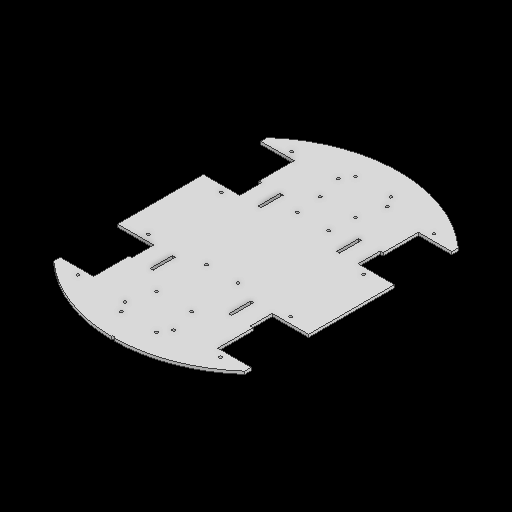
# Autodesk Inventor part: ChasisInferior
Saved by Autodesk Inventor 2025.2 (Build 292293000, 293)
## iProperties
Created: 2024-12-02
Part Number: ChasisInferior
Material: Generic
Document SubType Name: Modeling
Designer: braughton
Density: 1 g/cm^3
Appearance: Default
Author: braughton
Autodesk Inventor part; units mm, degrees
ref_plane "YZ Plane" through (0, 0, 0) normal (1, 0, 0) x (0, 1, 0)
ref_plane "XZ Plane" through (0, 0, 0) normal (0, 1, 0) x (-1, 0, 0)
ref_plane "XY Plane" through (0, 0, 0) normal (0, 0, 1) x (1, 0, 0)
sketch "Sketch1" plane through (0, 0, 0) normal (0, 1, 0) x (-1, 0, 0)
  circle A0 centre (-19.704, -123.7953) radius 1.5
  circle A1 centre (-26.6684, -112.9171) radius 1.5
  circle A2 centre (-75.7396, -112.9171) radius 1.5
  line L0 (-101.204, -106.1137) -> (-89.704, -106.1137)
  line L1 (-101.204, -106.1137) -> (-66.204, -106.1137)
  arc A3 (-101.204, -112.9171) -> (-1.204, -151.1137) centre (-1.204, -1.1137) ccw
  line L2 (-101.204, -106.1137) -> (-101.204, -112.9171)
  line L3 (-89.704, -106.1137) -> (-78.204, -106.1137)
  circle A4 centre (17.296, 121.5679) radius 1.5
  circle A5 centre (17.296, 84.5679) radius 1.5
  line L4 (63.796, 103.8863) -> (63.796, 66.8863)
  circle A6 centre (24.2604, 110.6897) radius 1.5
  circle A7 centre (73.3316, 110.6897) radius 1.5
  line L5 (98.796, 103.8863) -> (63.796, 103.8863)
  arc A8 (98.796, 110.6897) -> (-1.204, 148.8863) centre (-1.204, -1.1137) ccw
  line L6 (75.796, 43.8863) -> (87.296, 43.8863)
  circle A9 centre (73.3316, 37.0829) radius 1.5
  line L7 (87.296, 43.8863) -> (98.796, 43.8863)
  circle A10 centre (-19.704, 121.5679) radius 1.5
  circle A11 centre (-1.204, 148.8863) radius 1.5
  circle A12 centre (-26.6684, 110.6897) radius 1.5
  circle A13 centre (-75.7396, 110.6897) radius 1.5
  line L8 (-101.204, 103.8863) -> (-66.204, 103.8863)
  line L9 (-101.204, 103.8863) -> (-101.204, 110.6897)
  arc A14 (-1.204, 148.8863) -> (-101.204, 110.6897) centre (-1.204, -1.1137) ccw
  line L10 (-2.704, 148.8863) -> (-1.204, 148.8863)
  line L11 (0.296, 148.8863) -> (-1.204, 148.8863)
  line L12 (63.796, -69.1137) -> (60.796, -69.1137)
  line L13 (38.396, -69.1137) -> (41.396, -69.1137)
  line L14 (63.796, -46.1137) -> (98.796, -46.1137)
  line L15 (60.796, -69.1137) -> (60.796, -57.6137)
  line L16 (41.396, -69.1137) -> (41.396, -57.6137)
  line L17 (63.796, -46.1137) -> (60.796, -46.1137)
  line L18 (60.796, -46.1137) -> (60.796, -57.6137)
  line L19 (41.396, -46.1137) -> (41.396, -57.6137)
  line L20 (38.396, -46.1137) -> (41.396, -46.1137)
  line L21 (38.396, -57.6137) -> (38.396, -46.1137)
  circle A15 centre (73.3316, -39.3103) radius 1.5
  line L22 (38.396, -57.6137) -> (38.396, -69.1137)
  circle A16 centre (17.296, -123.7953) radius 1.5
  circle A17 centre (17.296, -86.7953) radius 1.5
  circle A18 centre (15.296, -60.7953) radius 1.5
  line L23 (75.796, -106.1137) -> (87.296, -106.1137)
  line L24 (87.296, -106.1137) -> (98.796, -106.1137)
  circle A19 centre (24.2604, -112.9171) radius 1.5
  line L25 (63.796, -106.1137) -> (63.796, -69.1137)
  circle A20 centre (73.3316, -112.9171) radius 1.5
  arc A21 (-1.204, -151.1137) -> (98.796, -112.9171) centre (-1.204, -1.1137) ccw
  line L26 (98.796, -106.1137) -> (63.796, -106.1137)
  circle A22 centre (-17.704, 34.2047) radius 1.5
  line L27 (-101.204, 43.8863) -> (-89.704, 43.8863)
  line L28 (-89.704, 43.8863) -> (-78.204, 43.8863)
  circle A23 centre (-75.7396, 37.0829) radius 1.5
  circle A24 centre (-75.7396, -39.3103) radius 1.5
  line L29 (-66.204, -46.1137) -> (-101.204, -46.1137)
  line L30 (-66.204, 43.8863) -> (-101.204, 43.8863)
  line L31 (-66.204, -46.1137) -> (-63.204, -46.1137)
  line L32 (-101.204, -1.1137) -> (-101.204, -46.1137)
  line L33 (-101.204, -1.1137) -> (-101.204, 43.8863)
  line L34 (98.796, -1.1137) -> (98.796, -46.1137)
  line L35 (98.796, -1.1137) -> (98.796, -46.1137)
  line L36 (98.796, -1.1137) -> (98.796, 43.8863)
  line L37 (98.796, -1.1137) -> (98.796, 43.8863)
  circle A25 centre (-19.704, 84.5679) radius 1.5
  line L38 (-66.204, 103.8863) -> (-66.204, 66.8863)
  line L39 (-40.804, 66.8863) -> (-43.804, 66.8863)
  line L40 (-40.804, 55.3863) -> (-40.804, 66.8863)
  line L41 (-43.804, 66.8863) -> (-43.804, 55.3863)
  line L42 (-66.204, 66.8863) -> (-63.204, 66.8863)
  line L43 (-63.204, 66.8863) -> (-63.204, 55.3863)
  line L44 (-40.804, 55.3863) -> (-40.804, 43.8863)
  line L45 (-40.804, 43.8863) -> (-43.804, 43.8863)
  line L46 (-43.804, 43.8863) -> (-43.804, 55.3863)
  line L47 (-63.204, 43.8863) -> (-63.204, 55.3863)
  line L48 (-66.204, 43.8863) -> (-63.204, 43.8863)
  circle A26 centre (-19.704, -86.7953) radius 1.5
  line L49 (-66.204, -106.1137) -> (-66.204, -69.1137)
  line L50 (-66.204, -69.1137) -> (-63.204, -69.1137)
  line L51 (-40.804, -69.1137) -> (-43.804, -69.1137)
  line L52 (-43.804, -69.1137) -> (-43.804, -57.6137)
  line L53 (-40.804, -57.6137) -> (-40.804, -69.1137)
  line L54 (-63.204, -46.1137) -> (-63.204, -57.6137)
  circle A27 centre (-17.704, -60.7953) radius 1.5
  line L55 (-43.804, -46.1137) -> (-43.804, -57.6137)
  line L56 (-40.804, -46.1137) -> (-43.804, -46.1137)
  line L57 (-40.804, -57.6137) -> (-40.804, -46.1137)
  line L58 (-63.204, -69.1137) -> (-63.204, -57.6137)
  line L59 (98.796, 103.8863) -> (98.796, 110.6897)
  line L60 (98.796, 103.8863) -> (98.796, 110.6897)
  line L61 (98.796, -106.1137) -> (98.796, -112.9171)
  line L62 (98.796, -106.1137) -> (98.796, -112.9171)
  line L63 (63.796, 43.8863) -> (98.796, 43.8863)
  line L64 (63.796, 66.8863) -> (60.796, 66.8863)
  line L65 (38.396, 66.8863) -> (41.396, 66.8863)
  line L66 (60.796, 66.8863) -> (60.796, 55.3863)
  line L67 (41.396, 66.8863) -> (41.396, 55.3863)
  line L68 (38.396, 55.3863) -> (38.396, 66.8863)
  line L69 (63.796, 43.8863) -> (60.796, 43.8863)
  line L70 (60.796, 43.8863) -> (60.796, 55.3863)
  line L71 (41.396, 43.8863) -> (41.396, 55.3863)
  line L72 (38.396, 43.8863) -> (41.396, 43.8863)
  line L73 (38.396, 55.3863) -> (38.396, 43.8863)
  circle A28 centre (15.296, 34.2047) radius 1.5
  point P0 (0, 0)
  point P1 (0.296, 148.8863)
  point P2 (-2.704, 148.8788)
  constraints: 148 end point, 29 centre point, 10 point on circle, 8 point on line
extrude "Extrusion1" add sketch "Sketch1" along normal blind 3 contours L0 L1 L49 L50 L58 L54 L31 L29 L32 L33 L27 L28 L30 L48 L47 L43 L42 L38 L8 L9 A14 A11 A8 L59 L5 L4 L64 L66 L70 L69 L63 L6 L7 L36 L34 L14 L17 L18 L15 L12 L25 L26 L23 L24 L61 A21 A3 L2
body "Solid1"
